Autodesk Inventor part; units mm, degrees
(part 2 of 2)
  line L281 (-95.3704, -44.7498) -> (-95.3704, -45.6606)
  spline S232 degree 2 poles (-95.3704, -45.6606) (-95.3704, -46.2246) (-95.539, -46.8665) (-95.6881, -47.0934) knots 0 0 0 1 2 2 2
  spline S233 degree 2 poles (-95.6881, -47.0934) (-95.9442, -47.4791) (-96.7902, -47.9037) (-97.3737, -47.9037) knots 0 0 0 1 2 2 2
  spline S234 degree 2 poles (-97.3672, -47.3494) (-96.9069, -47.3494) (-96.2553, -47.0447) (-96.0706, -46.7433) knots 0 0 0 1 2 2 2
  spline S235 degree 2 poles (-96.0706, -46.7433) (-95.9442, -46.5293) (-95.8307, -46.0464) (-95.8307, -45.6866) knots 0 0 0 1 2 2 2
  line L282 (-95.8307, -45.6866) -> (-95.8307, -45.2814)
  line L283 (-95.8307, -45.2814) -> (-98.9101, -45.2814)
  line L284 (-98.9101, -45.2814) -> (-98.9101, -45.6866)
  spline S236 degree 2 poles (-98.9101, -45.6866) (-98.9101, -46.0399) (-98.7967, -46.5747) (-98.6443, -46.7919) knots 0 0 0 1 2 2 2
  spline S237 degree 2 poles (-98.6443, -46.7919) (-98.4563, -47.0707) (-97.8339, -47.3494) (-97.3672, -47.3494) knots 0 0 0 1 2 2 2
  spline S238 degree 2 poles (-99.4385, -49.7449) (-99.4385, -49.0253) (-98.6314, -48.2344) (-97.8858, -48.2344) knots 0 0 0 1 2 2 2
  spline S239 degree 2 poles (-97.8858, -48.2344) (-97.1532, -48.2344) (-96.2845, -49.0026) (-96.2845, -49.6217) knots 0 0 0 1 2 2 2
  spline S240 degree 2 poles (-96.2845, -49.6217) (-96.2845, -49.9005) (-96.4466, -50.3316) (-96.6184, -50.4904) knots 0 0 0 1 2 2 2
  spline S241 degree 2 poles (-96.6184, -50.4904) (-96.7902, -50.6525) (-97.2861, -50.8243) (-97.6459, -50.8243) knots 0 0 0 1 2 2 2
  line L285 (-97.6459, -50.8243) -> (-97.9215, -50.8243)
  line L286 (-97.9215, -50.8243) -> (-97.9215, -48.7465)
  spline S242 degree 2 poles (-97.9215, -48.7465) (-98.4433, -48.7465) (-98.9976, -49.2716) (-98.9976, -49.7384) knots 0 0 0 1 2 2 2
  spline S243 degree 2 poles (-98.9976, -49.7384) (-98.9976, -49.9037) (-98.9231, -50.2246) (-98.8647, -50.3543) knots 0 0 0 1 2 2 2
  spline S244 degree 2 poles (-98.8647, -50.3543) (-98.7999, -50.4904) (-98.6865, -50.6784) (-98.6346, -50.74) knots 0 0 0 1 2 2 2
  line L287 (-98.6346, -50.74) -> (-98.6346, -50.7692)
  line L288 (-98.6346, -50.7692) -> (-99.1856, -50.7692)
  spline S245 degree 2 poles (-99.1856, -50.7692) (-99.2213, -50.6817) (-99.325, -50.4159) (-99.3542, -50.3122) knots 0 0 0 1 2 2 2
  spline S246 degree 2 poles (-99.3542, -50.3122) (-99.3963, -50.1663) (-99.4385, -49.9264) (-99.4385, -49.7449) knots 0 0 0 1 2 2 2
  spline S247 degree 2 poles (-97.5357, -50.3316) (-97.3315, -50.3251) (-97.0333, -50.2408) (-96.9328, -50.1598) knots 0 0 0 1 2 2 2
  spline S248 degree 2 poles (-96.9328, -50.1598) (-96.8194, -50.0723) (-96.6994, -49.7968) (-96.6994, -49.5926) knots 0 0 0 1 2 2 2
  spline S249 degree 2 poles (-96.6994, -49.5926) (-96.6994, -49.3916) (-96.8194, -49.1096) (-96.9361, -48.9929) knots 0 0 0 1 2 2 2
  spline S250 degree 2 poles (-96.9361, -48.9929) (-97.056, -48.8794) (-97.3445, -48.7627) (-97.5357, -48.7465) knots 0 0 0 1 2 2 2
  line L289 (-97.5357, -48.7465) -> (-97.5357, -50.3316)
  spline S251 degree 2 poles (-99.4417, -52.1468) (-99.4417, -51.8454) (-99.2797, -51.3235) (-99.1889, -51.1517) knots 0 0 0 1 2 2 2
  line L290 (-99.1889, -51.1517) -> (-98.6216, -51.1517)
  line L291 (-98.6216, -51.1517) -> (-98.6216, -51.1776)
  spline S252 degree 2 poles (-98.6216, -51.1776) (-98.6735, -51.2425) (-98.7967, -51.4175) (-98.8647, -51.5634) knots 0 0 0 1 2 2 2
  spline S253 degree 2 poles (-98.8647, -51.5634) (-98.9263, -51.6898) (-99.0171, -52.001) (-99.0171, -52.1663) knots 0 0 0 1 2 2 2
  spline S254 degree 2 poles (-99.0171, -52.1663) (-99.0171, -52.2862) (-98.962, -52.5618) (-98.9166, -52.6266) knots 0 0 0 1 2 2 2
  spline S255 degree 2 poles (-98.9166, -52.6266) (-98.855, -52.7206) (-98.7156, -52.8049) (-98.573, -52.8049) knots 0 0 0 1 2 2 2
  spline S256 degree 2 poles (-98.573, -52.8049) (-98.3947, -52.8049) (-98.21, -52.6104) (-98.1484, -52.3608) knots 0 0 0 1 2 2 2
  spline S257 degree 2 poles (-98.1484, -52.3608) (-98.1257, -52.2635) (-98.0609, -51.9524) (-98.0252, -51.8195) knots 0 0 0 1 2 2 2
  spline S258 degree 2 poles (-98.0252, -51.8195) (-97.9247, -51.4759) (-97.5098, -51.1647) (-97.2148, -51.1647) knots 0 0 0 1 2 2 2
  spline S259 degree 2 poles (-97.2148, -51.1647) (-96.8064, -51.1647) (-96.2975, -51.7773) (-96.2975, -52.283) knots 0 0 0 1 2 2 2
  spline S260 degree 2 poles (-96.2975, -52.283) (-96.2975, -52.5326) (-96.4207, -53.0383) (-96.5147, -53.2101) knots 0 0 0 1 2 2 2
  line L292 (-96.5147, -53.2101) -> (-97.056, -53.2101)
  line L293 (-97.056, -53.2101) -> (-97.056, -53.1841)
  spline S261 degree 2 poles (-97.056, -53.1841) (-96.9004, -52.9896) (-96.7221, -52.5164) (-96.7221, -52.2733) knots 0 0 0 1 2 2 2
  spline S262 degree 2 poles (-96.7221, -52.2733) (-96.7221, -52.0237) (-96.9328, -51.6801) (-97.1435, -51.6801) knots 0 0 0 1 2 2 2
  spline S263 degree 2 poles (-97.1435, -51.6801) (-97.3348, -51.6801) (-97.5195, -51.8843) (-97.5779, -52.1112) knots 0 0 0 1 2 2 2
  spline S264 degree 2 poles (-97.5779, -52.1112) (-97.607, -52.2214) (-97.6654, -52.5002) (-97.701, -52.6525) knots 0 0 0 1 2 2 2
  spline S265 degree 2 poles (-97.701, -52.6525) (-97.7853, -52.9831) (-98.1711, -53.3203) (-98.5049, -53.3203) knots 0 0 0 1 2 2 2
  spline S266 degree 2 poles (-98.5049, -53.3203) (-98.6994, -53.3203) (-99.043, -53.1679) (-99.1694, -53.0188) knots 0 0 0 1 2 2 2
  spline S267 degree 2 poles (-99.1694, -53.0188) (-99.3023, -52.86) (-99.4417, -52.4548) (-99.4417, -52.1468) knots 0 0 0 1 2 2 2
  line L294 (-99.3704, -54.3057) -> (-99.3704, -53.8)
  line L295 (-99.3704, -53.8) -> (-96.3688, -53.8)
  line L296 (-96.3688, -53.8) -> (-96.3688, -54.3057)
  line L297 (-96.3688, -54.3057) -> (-99.3704, -54.3057)
  line L298 (-95.8696, -54.3413) -> (-95.8696, -53.7676)
  line L299 (-95.8696, -53.7676) -> (-95.3445, -53.7676)
  line L300 (-95.3445, -53.7676) -> (-95.3445, -54.3413)
  line L301 (-95.3445, -54.3413) -> (-95.8696, -54.3413)
  spline S268 degree 2 poles (-99.8502, -55.1549) (-99.8728, -55.2068) (-99.9442, -55.4045) (-99.9733, -55.531) knots 0 0 0 1 2 2 2
  spline S269 degree 2 poles (-99.9733, -55.531) (-100.009, -55.6703) (-100.0511, -55.907) (-100.0511, -56.0464) knots 0 0 0 1 2 2 2
  spline S270 degree 2 poles (-100.0511, -56.0464) (-100.0511, -56.2797) (-99.9279, -56.6039) (-99.8177, -56.6947) knots 0 0 0 1 2 2 2
  spline S271 degree 2 poles (-99.8177, -56.6947) (-99.7075, -56.7822) (-99.419, -56.8502) (-99.2343, -56.8502) knots 0 0 0 1 2 2 2
  line L302 (-99.2343, -56.8502) -> (-98.9717, -56.8502)
  spline S272 degree 2 poles (-98.9717, -56.8502) (-99.15, -56.646) (-99.3185, -56.2538) (-99.3185, -55.9588) knots 0 0 0 1 2 2 2
  spline S273 degree 2 poles (-99.3185, -55.9588) (-99.3185, -55.4467) (-98.5568, -54.8405) (-97.8404, -54.8405) knots 0 0 0 1 2 2 2
  spline S274 degree 2 poles (-97.8404, -54.8405) (-97.4677, -54.8405) (-96.8907, -55.0512) (-96.6865, -55.2263) knots 0 0 0 1 2 2 2
  spline S275 degree 2 poles (-96.6865, -55.2263) (-96.4952, -55.3948) (-96.2845, -55.8584) (-96.2845, -56.1047) knots 0 0 0 1 2 2 2
  spline S276 degree 2 poles (-96.2845, -56.1047) (-96.2845, -56.3381) (-96.3947, -56.6784) (-96.4952, -56.8502) knots 0 0 0 1 2 2 2
  line L303 (-96.4952, -56.8502) -> (-96.3688, -56.8794)
  line L304 (-96.3688, -56.8794) -> (-96.3688, -57.3559)
  line L305 (-96.3688, -57.3559) -> (-99.0268, -57.3559)
  spline S277 degree 2 poles (-99.0268, -57.3559) (-99.7918, -57.3559) (-100.5049, -56.6914) (-100.5049, -56.0075) knots 0 0 0 1 2 2 2
  spline S278 degree 2 poles (-100.5049, -56.0075) (-100.5049, -55.787) (-100.4336, -55.3267) (-100.3753, -55.129) knots 0 0 0 1 2 2 2
  line L306 (-100.3753, -55.129) -> (-99.8502, -55.129)
  line L307 (-99.8502, -55.129) -> (-99.8502, -55.1549)
  line L308 (-98.5568, -56.8502) -> (-96.9069, -56.8502)
  spline S279 degree 2 poles (-96.9069, -56.8502) (-96.8161, -56.6622) (-96.7383, -56.3446) (-96.7383, -56.1857) knots 0 0 0 1 2 2 2
  spline S280 degree 2 poles (-96.7383, -56.1857) (-96.7383, -55.8032) (-97.3023, -55.3624) (-97.8307, -55.3624) knots 0 0 0 1 2 2 2
  spline S281 degree 2 poles (-97.8307, -55.3624) (-98.3299, -55.3624) (-98.8518, -55.6963) (-98.8518, -56.0723) knots 0 0 0 1 2 2 2
  spline S282 degree 2 poles (-98.8518, -56.0723) (-98.8518, -56.27) (-98.6962, -56.6849) (-98.5568, -56.8502) knots 0 0 0 1 2 2 2
  line L309 (-99.3704, -60.4451) -> (-99.3704, -59.9394)
  line L310 (-99.3704, -59.9394) -> (-97.6589, -59.9394)
  spline S283 degree 2 poles (-97.6589, -59.9394) (-97.4514, -59.9394) (-97.0949, -59.9005) (-96.9879, -59.8421) knots 0 0 0 1 2 2 2
  spline S284 degree 2 poles (-96.9879, -59.8421) (-96.8745, -59.7806) (-96.7643, -59.5601) (-96.7643, -59.3721) knots 0 0 0 1 2 2 2
  spline S285 degree 2 poles (-96.7643, -59.3721) (-96.7643, -59.1841) (-96.9652, -58.7854) (-97.1273, -58.5942) knots 0 0 0 1 2 2 2
  line L311 (-97.1273, -58.5942) -> (-99.3704, -58.5942)
  line L312 (-99.3704, -58.5942) -> (-99.3704, -58.0885)
  line L313 (-99.3704, -58.0885) -> (-96.3688, -58.0885)
  line L314 (-96.3688, -58.0885) -> (-96.3688, -58.5942)
  line L315 (-96.3688, -58.5942) -> (-96.7027, -58.5942)
  spline S286 degree 2 poles (-96.7027, -58.5942) (-96.4985, -58.8211) (-96.2845, -59.2587) (-96.2845, -59.505) knots 0 0 0 1 2 2 2
  spline S287 degree 2 poles (-96.2845, -59.505) (-96.2845, -59.9459) (-96.868, -60.4451) (-97.4223, -60.4451) knots 0 0 0 1 2 2 2
  line L316 (-97.4223, -60.4451) -> (-99.3704, -60.4451)
  spline S288 degree 2 poles (-98.1419, -65.625) (-98.4401, -65.625) (-98.8972, -65.3981) (-99.0463, -65.2101) knots 0 0 0 1 2 2 2
  spline S289 degree 2 poles (-99.0463, -65.2101) (-99.2213, -64.9831) (-99.3704, -64.4678) (-99.3704, -64.0593) knots 0 0 0 1 2 2 2
  line L317 (-99.3704, -64.0593) -> (-99.3704, -62.9118)
  line L318 (-99.3704, -62.9118) -> (-95.3704, -62.9118)
  line L319 (-95.3704, -62.9118) -> (-95.3704, -63.9718)
  spline S290 degree 2 poles (-95.3704, -63.9718) (-95.3704, -64.3997) (-95.4255, -64.8276) (-95.5325, -65.022) knots 0 0 0 1 2 2 2
  spline S291 degree 2 poles (-95.5325, -65.022) (-95.6459, -65.2392) (-96.0187, -65.437) (-96.2715, -65.437) knots 0 0 0 1 2 2 2
  spline S292 degree 2 poles (-96.2715, -65.437) (-96.5536, -65.437) (-97.0009, -65.1387) (-97.1273, -64.8762) knots 0 0 0 1 2 2 2
  line L320 (-97.1273, -64.8762) -> (-97.1467, -64.8762)
  spline S293 degree 2 poles (-97.1467, -64.8762) (-97.244, -65.2327) (-97.7594, -65.625) (-98.1419, -65.625) knots 0 0 0 1 2 2 2
  spline S294 degree 2 poles (-98.1646, -65.0707) (-97.9377, -65.0707) (-97.6459, -64.941) (-97.5422, -64.7465) knots 0 0 0 1 2 2 2
  spline S295 degree 2 poles (-97.5422, -64.7465) (-97.4774, -64.6201) (-97.4385, -64.3219) (-97.4385, -64.0464) knots 0 0 0 1 2 2 2
  line L321 (-97.4385, -64.0464) -> (-97.4385, -63.4434)
  line L322 (-97.4385, -63.4434) -> (-98.9166, -63.4434)
  line L323 (-98.9166, -63.4434) -> (-98.9166, -63.8746)
  spline S296 degree 2 poles (-98.9166, -63.8746) (-98.9166, -64.2246) (-98.8518, -64.6266) (-98.748, -64.7822) knots 0 0 0 1 2 2 2
  spline S297 degree 2 poles (-98.748, -64.7822) (-98.6411, -64.9313) (-98.3753, -65.0707) (-98.1646, -65.0707) knots 0 0 0 1 2 2 2
  spline S298 degree 2 poles (-96.3461, -64.8827) (-96.2035, -64.8827) (-95.9895, -64.7854) (-95.9279, -64.6784) knots 0 0 0 1 2 2 2
  spline S299 degree 2 poles (-95.9279, -64.6784) (-95.8566, -64.5488) (-95.8242, -64.2344) (-95.8242, -63.9524) knots 0 0 0 1 2 2 2
  line L324 (-95.8242, -63.9524) -> (-95.8242, -63.4434)
  line L325 (-95.8242, -63.4434) -> (-96.9944, -63.4434)
  line L326 (-96.9944, -63.4434) -> (-96.9944, -64.0464)
  spline S300 degree 2 poles (-96.9944, -64.0464) (-96.9944, -64.296) (-96.9425, -64.5326) (-96.8615, -64.659) knots 0 0 0 1 2 2 2
  spline S301 degree 2 poles (-96.8615, -64.659) (-96.7837, -64.7822) (-96.5341, -64.8827) (-96.3461, -64.8827) knots 0 0 0 1 2 2 2
  line L327 (-96.3688, -68.471) -> (-100.4758, -66.8567)
  line L328 (-100.4758, -66.8567) -> (-100.4758, -66.3154)
  line L329 (-100.4758, -66.3154) -> (-99.2245, -66.8535)
  line L330 (-99.2245, -66.8535) -> (-96.3688, -65.7643)
  line L331 (-96.3688, -65.7643) -> (-96.3688, -66.3089)
  line L332 (-96.3688, -66.3089) -> (-98.5925, -67.129)
  line L333 (-98.5925, -67.129) -> (-96.3688, -67.9459)
  line L334 (-96.3688, -67.9459) -> (-96.3688, -68.471)
  line L335 (-99.3704, -69.7806) -> (-99.3704, -69.1387)
  line L336 (-99.3704, -69.1387) -> (-98.6054, -69.1387)
  line L337 (-98.6054, -69.1387) -> (-98.6054, -69.7806)
  line L338 (-98.6054, -69.7806) -> (-99.3704, -69.7806)
  line L339 (-97.1338, -69.7806) -> (-97.1338, -69.1387)
  line L340 (-97.1338, -69.1387) -> (-96.3688, -69.1387)
  line L341 (-96.3688, -69.1387) -> (-96.3688, -69.7806)
  line L342 (-96.3688, -69.7806) -> (-97.1338, -69.7806)
  line L343 (-109.2392, -46.2221) -> (-109.2392, -44.2853)
  line L344 (-109.2392, -44.2853) -> (-108.7287, -44.2853)
  line L345 (-108.7287, -44.2853) -> (-108.7287, -44.9215)
  line L346 (-108.7287, -44.9215) -> (-104.7498, -44.9215)
  line L347 (-104.7498, -44.9215) -> (-104.7498, -44.2853)
  line L348 (-104.7498, -44.2853) -> (-104.2392, -44.2853)
  line L349 (-104.2392, -44.2853) -> (-104.2392, -46.2221)
  line L350 (-104.2392, -46.2221) -> (-104.7498, -46.2221)
  line L351 (-104.7498, -46.2221) -> (-104.7498, -45.586)
  line L352 (-104.7498, -45.586) -> (-108.7287, -45.586)
  line L353 (-108.7287, -45.586) -> (-108.7287, -46.2221)
  line L354 (-108.7287, -46.2221) -> (-109.2392, -46.2221)
  line L355 (-109.2392, -51.2505) -> (-107.0674, -51.2505)
  spline S302 degree 2 poles (-107.0674, -51.2505) (-106.8081, -51.2505) (-106.3665, -51.21) (-106.2449, -51.1451) knots 0 0 0 1 2 2 2
  spline S303 degree 2 poles (-106.2449, -51.1451) (-106.1112, -51.0803) (-105.9815, -50.8331) (-105.9815, -50.6184) knots 0 0 0 1 2 2 2
  spline S304 degree 2 poles (-105.9815, -50.6184) (-105.9815, -50.4239) (-106.2206, -49.9782) (-106.4475, -49.7432) knots 0 0 0 1 2 2 2
  spline S305 degree 2 poles (-106.4475, -49.7432) (-106.5042, -49.7472) (-106.6622, -49.7553) (-106.7676, -49.7553) knots 0 0 0 1 2 2 2
  line L356 (-106.7676, -49.7553) -> (-109.2392, -49.7553)
  line L357 (-109.2392, -49.7553) -> (-109.2392, -49.1232)
  line L358 (-109.2392, -49.1232) -> (-107.0674, -49.1232)
  spline S306 degree 2 poles (-107.0674, -49.1232) (-106.8081, -49.1232) (-106.3665, -49.0827) (-106.2449, -49.0179) knots 0 0 0 1 2 2 2
  spline S307 degree 2 poles (-106.2449, -49.0179) (-106.1112, -48.9531) (-105.9815, -48.7059) (-105.9815, -48.4912) knots 0 0 0 1 2 2 2
  spline S308 degree 2 poles (-105.9815, -48.4912) (-105.9815, -48.2886) (-106.2368, -47.8388) (-106.4353, -47.6281) knots 0 0 0 1 2 2 2
  line L359 (-106.4353, -47.6281) -> (-109.2392, -47.6281)
  line L360 (-109.2392, -47.6281) -> (-109.2392, -46.996)
  line L361 (-109.2392, -46.996) -> (-105.4872, -46.996)
  line L362 (-105.4872, -46.996) -> (-105.4872, -47.6281)
  line L363 (-105.4872, -47.6281) -> (-105.9005, -47.6281)
  spline S309 degree 2 poles (-105.9005, -47.6281) (-105.6533, -47.8753) (-105.3819, -48.3615) (-105.3819, -48.6532) knots 0 0 0 1 2 2 2
  spline S310 degree 2 poles (-105.3819, -48.6532) (-105.3819, -48.9855) (-105.6857, -49.5001) (-106.0302, -49.6338) knots 0 0 0 1 2 2 2
  spline S311 degree 2 poles (-106.0302, -49.6338) (-105.7101, -49.9215) (-105.3819, -50.4644) (-105.3819, -50.7805) knots 0 0 0 1 2 2 2
  spline S312 degree 2 poles (-105.3819, -50.7805) (-105.3819, -51.0236) (-105.5318, -51.4207) (-105.702, -51.5665) knots 0 0 0 1 2 2 2
  spline S313 degree 2 poles (-105.702, -51.5665) (-105.8721, -51.7164) (-106.3827, -51.8826) (-106.7676, -51.8826) knots 0 0 0 1 2 2 2
  line L364 (-106.7676, -51.8826) -> (-109.2392, -51.8826)
  line L365 (-109.2392, -51.8826) -> (-109.2392, -51.2505)
  spline S314 degree 2 poles (-107.3632, -55.8534) (-108.3114, -55.8534) (-109.3446, -54.9417) (-109.3446, -54.18) knots 0 0 0 1 2 2 2
  spline S315 degree 2 poles (-109.3446, -54.18) (-109.3446, -53.398) (-108.2789, -52.5025) (-107.3632, -52.5025) knots 0 0 0 1 2 2 2
  spline S316 degree 2 poles (-107.3632, -52.5025) (-106.4232, -52.5025) (-105.3819, -53.4263) (-105.3819, -54.18) knots 0 0 0 1 2 2 2
  spline S317 degree 2 poles (-105.3819, -54.18) (-105.3819, -54.9417) (-106.4191, -55.8534) (-107.3632, -55.8534) knots 0 0 0 1 2 2 2
  spline S318 degree 2 poles (-107.3632, -55.201) (-106.6339, -55.201) (-105.9248, -54.6703) (-105.9248, -54.18) knots 0 0 0 1 2 2 2
  spline S319 degree 2 poles (-105.9248, -54.18) (-105.9248, -53.6897) (-106.6339, -53.1549) (-107.3632, -53.1549) knots 0 0 0 1 2 2 2
  spline S320 degree 2 poles (-107.3632, -53.1549) (-108.0723, -53.1549) (-108.8016, -53.6897) (-108.8016, -54.18) knots 0 0 0 1 2 2 2
  spline S321 degree 2 poles (-108.8016, -54.18) (-108.8016, -54.6662) (-108.0845, -55.201) (-107.3632, -55.201) knots 0 0 0 1 2 2 2
  spline S322 degree 2 poles (-109.8389, -56.6354) (-109.8673, -56.7002) (-109.9564, -56.9474) (-109.9929, -57.1054) knots 0 0 0 1 2 2 2
  spline S323 degree 2 poles (-109.9929, -57.1054) (-110.0375, -57.2797) (-110.0901, -57.5754) (-110.0901, -57.7497) knots 0 0 0 1 2 2 2
  spline S324 degree 2 poles (-110.0901, -57.7497) (-110.0901, -58.0414) (-109.9362, -58.4466) (-109.7984, -58.56) knots 0 0 0 1 2 2 2
  spline S325 degree 2 poles (-109.7984, -58.56) (-109.6606, -58.6694) (-109.3, -58.7545) (-109.0691, -58.7545) knots 0 0 0 1 2 2 2
  line L366 (-109.0691, -58.7545) -> (-108.7409, -58.7545)
  spline S326 degree 2 poles (-108.7409, -58.7545) (-108.9637, -58.4993) (-109.1744, -58.009) (-109.1744, -57.6403) knots 0 0 0 1 2 2 2
  spline S327 degree 2 poles (-109.1744, -57.6403) (-109.1744, -57.0001) (-108.2222, -56.2424) (-107.3268, -56.2424) knots 0 0 0 1 2 2 2
  spline S328 degree 2 poles (-107.3268, -56.2424) (-106.8608, -56.2424) (-106.1396, -56.5057) (-105.8843, -56.7245) knots 0 0 0 1 2 2 2
  spline S329 degree 2 poles (-105.8843, -56.7245) (-105.6452, -56.9352) (-105.3819, -57.5147) (-105.3819, -57.8226) knots 0 0 0 1 2 2 2
  spline S330 degree 2 poles (-105.3819, -57.8226) (-105.3819, -58.1143) (-105.5196, -58.5398) (-105.6452, -58.7545) knots 0 0 0 1 2 2 2
  line L367 (-105.6452, -58.7545) -> (-105.4872, -58.791)
  line L368 (-105.4872, -58.791) -> (-105.4872, -59.3866)
  line L369 (-105.4872, -59.3866) -> (-108.8097, -59.3866)
  spline S331 degree 2 poles (-108.8097, -59.3866) (-109.766, -59.3866) (-110.6574, -58.556) (-110.6574, -57.701) knots 0 0 0 1 2 2 2
  spline S332 degree 2 poles (-110.6574, -57.701) (-110.6574, -57.4255) (-110.5682, -56.8502) (-110.4953, -56.603) knots 0 0 0 1 2 2 2
  line L370 (-110.4953, -56.603) -> (-109.8389, -56.603)
  line L371 (-109.8389, -56.603) -> (-109.8389, -56.6354)
  line L372 (-108.2222, -58.7545) -> (-106.1598, -58.7545)
  spline S333 degree 2 poles (-106.1598, -58.7545) (-106.0464, -58.5195) (-105.9491, -58.1224) (-105.9491, -57.9239) knots 0 0 0 1 2 2 2
  spline S334 degree 2 poles (-105.9491, -57.9239) (-105.9491, -57.4458) (-106.6541, -56.8947) (-107.3146, -56.8947) knots 0 0 0 1 2 2 2
  spline S335 degree 2 poles (-107.3146, -56.8947) (-107.9386, -56.8947) (-108.5909, -57.3121) (-108.5909, -57.7821) knots 0 0 0 1 2 2 2
  spline S336 degree 2 poles (-108.5909, -57.7821) (-108.5909, -58.0292) (-108.3964, -58.5479) (-108.2222, -58.7545) knots 0 0 0 1 2 2 2
  spline S337 degree 2 poles (-109.3243, -61.9312) (-109.3243, -61.0317) (-108.3154, -60.043) (-107.3835, -60.043) knots 0 0 0 1 2 2 2
  spline S338 degree 2 poles (-107.3835, -60.043) (-106.4678, -60.043) (-105.3819, -61.0033) (-105.3819, -61.7772) knots 0 0 0 1 2 2 2
  spline S339 degree 2 poles (-105.3819, -61.7772) (-105.3819, -62.1257) (-105.5845, -62.6646) (-105.7992, -62.8631) knots 0 0 0 1 2 2 2
  spline S340 degree 2 poles (-105.7992, -62.8631) (-106.014, -63.0657) (-106.6339, -63.2805) (-107.0836, -63.2805) knots 0 0 0 1 2 2 2
  line L373 (-107.0836, -63.2805) -> (-107.4281, -63.2805)
  line L374 (-107.4281, -63.2805) -> (-107.4281, -60.6832)
  spline S341 degree 2 poles (-107.4281, -60.6832) (-108.0804, -60.6832) (-108.7733, -61.3396) (-108.7733, -61.9231) knots 0 0 0 1 2 2 2
  spline S342 degree 2 poles (-108.7733, -61.9231) (-108.7733, -62.1297) (-108.6801, -62.5309) (-108.6071, -62.6929) knots 0 0 0 1 2 2 2
  spline S343 degree 2 poles (-108.6071, -62.6929) (-108.5261, -62.8631) (-108.3843, -63.0981) (-108.3195, -63.1751) knots 0 0 0 1 2 2 2
  line L375 (-108.3195, -63.1751) -> (-108.3195, -63.2116)
  line L376 (-108.3195, -63.2116) -> (-109.0083, -63.2116)
  spline S344 degree 2 poles (-109.0083, -63.2116) (-109.0528, -63.1022) (-109.1825, -62.7699) (-109.219, -62.6403) knots 0 0 0 1 2 2 2
  spline S345 degree 2 poles (-109.219, -62.6403) (-109.2716, -62.4579) (-109.3243, -62.1581) (-109.3243, -61.9312) knots 0 0 0 1 2 2 2
  spline S346 degree 2 poles (-106.9459, -62.6646) (-106.6906, -62.6565) (-106.3178, -62.5511) (-106.1922, -62.4498) knots 0 0 0 1 2 2 2
  spline S347 degree 2 poles (-106.1922, -62.4498) (-106.0504, -62.3404) (-105.9005, -61.996) (-105.9005, -61.7408) knots 0 0 0 1 2 2 2
  spline S348 degree 2 poles (-105.9005, -61.7408) (-105.9005, -61.4895) (-106.0504, -61.137) (-106.1963, -60.9912) knots 0 0 0 1 2 2 2
  spline S349 degree 2 poles (-106.1963, -60.9912) (-106.3462, -60.8493) (-106.7068, -60.7035) (-106.9459, -60.6832) knots 0 0 0 1 2 2 2
  line L377 (-106.9459, -60.6832) -> (-106.9459, -62.6646)
  line L378 (-109.2392, -66.8664) -> (-109.2392, -66.2343)
  line L379 (-109.2392, -66.2343) -> (-107.0999, -66.2343)
  spline S350 degree 2 poles (-107.0999, -66.2343) (-106.8405, -66.2343) (-106.3948, -66.1856) (-106.2611, -66.1127) knots 0 0 0 1 2 2 2
  spline S351 degree 2 poles (-106.2611, -66.1127) (-106.1193, -66.0357) (-105.9815, -65.7602) (-105.9815, -65.5252) knots 0 0 0 1 2 2 2
  spline S352 degree 2 poles (-105.9815, -65.5252) (-105.9815, -65.2902) (-106.2328, -64.7918) (-106.4353, -64.5527) knots 0 0 0 1 2 2 2
  line L380 (-106.4353, -64.5527) -> (-109.2392, -64.5527)
  line L381 (-109.2392, -64.5527) -> (-109.2392, -63.9207)
  line L382 (-109.2392, -63.9207) -> (-105.4872, -63.9207)
  line L383 (-105.4872, -63.9207) -> (-105.4872, -64.5527)
  line L384 (-105.4872, -64.5527) -> (-105.9046, -64.5527)
  spline S353 degree 2 poles (-105.9046, -64.5527) (-105.6493, -64.8364) (-105.3819, -65.3834) (-105.3819, -65.6913) knots 0 0 0 1 2 2 2
  spline S354 degree 2 poles (-105.3819, -65.6913) (-105.3819, -66.2424) (-106.1112, -66.8664) (-106.8041, -66.8664) knots 0 0 0 1 2 2 2
  line L385 (-106.8041, -66.8664) -> (-109.2392, -66.8664)
  line L386 (-104.2392, -75.5536) -> (-109.2392, -74.2975)
  line L387 (-109.2392, -74.2975) -> (-109.2392, -73.5519)
  line L388 (-109.2392, -73.5519) -> (-105.0901, -72.5349)
  line L389 (-105.0901, -72.5349) -> (-109.2392, -71.5463)
  line L390 (-109.2392, -71.5463) -> (-109.2392, -70.8088)
  line L391 (-109.2392, -70.8088) -> (-104.2392, -69.5325)
  line L392 (-104.2392, -69.5325) -> (-104.2392, -70.2173)
  line L393 (-104.2392, -70.2173) -> (-108.3843, -71.2221)
  line L394 (-108.3843, -71.2221) -> (-104.2392, -72.2189)
  line L395 (-104.2392, -72.2189) -> (-104.2392, -72.8955)
  line L396 (-104.2392, -72.8955) -> (-108.4329, -73.9004)
  line L397 (-108.4329, -73.9004) -> (-104.2392, -74.9012)
  line L398 (-104.2392, -74.9012) -> (-104.2392, -75.5536)
  line L399 (-106.1639, -78.09) -> (-106.1639, -78.0576)
  spline S355 degree 2 poles (-106.1639, -78.0576) (-106.1436, -77.9847) (-106.1355, -77.8267) (-106.1355, -77.7173) knots 0 0 0 1 2 2 2
  spline S356 degree 2 poles (-106.1355, -77.7173) (-106.1355, -77.462) (-106.3584, -76.9596) (-106.5772, -76.7326) knots 0 0 0 1 2 2 2
  line L400 (-106.5772, -76.7326) -> (-109.2392, -76.7326)
  line L401 (-109.2392, -76.7326) -> (-109.2392, -76.1006)
  line L402 (-109.2392, -76.1006) -> (-105.4872, -76.1006)
  line L403 (-105.4872, -76.1006) -> (-105.4872, -76.7326)
  line L404 (-105.4872, -76.7326) -> (-106.0464, -76.7326)
  spline S357 degree 2 poles (-106.0464, -76.7326) (-105.7384, -77.0771) (-105.4872, -77.5916) (-105.4872, -77.8348) knots 0 0 0 1 2 2 2
  spline S358 degree 2 poles (-105.4872, -77.8348) (-105.4872, -77.932) (-105.4953, -78.0292) (-105.5075, -78.09) knots 0 0 0 1 2 2 2
  line L405 (-105.5075, -78.09) -> (-106.1639, -78.09)
  spline S359 degree 2 poles (-109.3243, -80.2091) (-109.3243, -79.3096) (-108.3154, -78.321) (-107.3835, -78.321) knots 0 0 0 1 2 2 2
  spline S360 degree 2 poles (-107.3835, -78.321) (-106.4678, -78.321) (-105.3819, -79.2813) (-105.3819, -80.0552) knots 0 0 0 1 2 2 2
  spline S361 degree 2 poles (-105.3819, -80.0552) (-105.3819, -80.4036) (-105.5845, -80.9425) (-105.7992, -81.1411) knots 0 0 0 1 2 2 2
  spline S362 degree 2 poles (-105.7992, -81.1411) (-106.014, -81.3437) (-106.6339, -81.5584) (-107.0836, -81.5584) knots 0 0 0 1 2 2 2
  line L406 (-107.0836, -81.5584) -> (-107.4281, -81.5584)
  line L407 (-107.4281, -81.5584) -> (-107.4281, -78.9612)
  spline S363 degree 2 poles (-107.4281, -78.9612) (-108.0804, -78.9612) (-108.7733, -79.6176) (-108.7733, -80.201) knots 0 0 0 1 2 2 2
  spline S364 degree 2 poles (-108.7733, -80.201) (-108.7733, -80.4077) (-108.6801, -80.8088) (-108.6071, -80.9709) knots 0 0 0 1 2 2 2
  spline S365 degree 2 poles (-108.6071, -80.9709) (-108.5261, -81.1411) (-108.3843, -81.3761) (-108.3195, -81.4531) knots 0 0 0 1 2 2 2
  line L408 (-108.3195, -81.4531) -> (-108.3195, -81.4895)
  line L409 (-108.3195, -81.4895) -> (-109.0083, -81.4895)
  spline S366 degree 2 poles (-109.0083, -81.4895) (-109.0528, -81.3801) (-109.1825, -81.0479) (-109.219, -80.9182) knots 0 0 0 1 2 2 2
  spline S367 degree 2 poles (-109.219, -80.9182) (-109.2716, -80.7359) (-109.3243, -80.4361) (-109.3243, -80.2091) knots 0 0 0 1 2 2 2
  spline S368 degree 2 poles (-106.9459, -80.9425) (-106.6906, -80.9344) (-106.3178, -80.8291) (-106.1922, -80.7278) knots 0 0 0 1 2 2 2
  spline S369 degree 2 poles (-106.1922, -80.7278) (-106.0504, -80.6184) (-105.9005, -80.274) (-105.9005, -80.0187) knots 0 0 0 1 2 2 2
  spline S370 degree 2 poles (-105.9005, -80.0187) (-105.9005, -79.7675) (-106.0504, -79.415) (-106.1963, -79.2691) knots 0 0 0 1 2 2 2
  spline S371 degree 2 poles (-106.1963, -79.2691) (-106.3462, -79.1273) (-106.7068, -78.9814) (-106.9459, -78.9612) knots 0 0 0 1 2 2 2
  line L410 (-106.9459, -78.9612) -> (-106.9459, -80.9425)
  line L411 (-109.2392, -85.1443) -> (-109.2392, -84.5122)
  line L412 (-109.2392, -84.5122) -> (-107.0999, -84.5122)
  spline S372 degree 2 poles (-107.0999, -84.5122) (-106.8405, -84.5122) (-106.3948, -84.4636) (-106.2611, -84.3907) knots 0 0 0 1 2 2 2
  spline S373 degree 2 poles (-106.2611, -84.3907) (-106.1193, -84.3137) (-105.9815, -84.0382) (-105.9815, -83.8032) knots 0 0 0 1 2 2 2
  spline S374 degree 2 poles (-105.9815, -83.8032) (-105.9815, -83.5681) (-106.2328, -83.0698) (-106.4353, -82.8307) knots 0 0 0 1 2 2 2
  line L413 (-106.4353, -82.8307) -> (-109.2392, -82.8307)
  line L414 (-109.2392, -82.8307) -> (-109.2392, -82.1986)
  line L415 (-109.2392, -82.1986) -> (-105.4872, -82.1986)
  line L416 (-105.4872, -82.1986) -> (-105.4872, -82.8307)
  line L417 (-105.4872, -82.8307) -> (-105.9046, -82.8307)
  spline S375 degree 2 poles (-105.9046, -82.8307) (-105.6493, -83.1143) (-105.3819, -83.6613) (-105.3819, -83.9693) knots 0 0 0 1 2 2 2
  spline S376 degree 2 poles (-105.3819, -83.9693) (-105.3819, -84.5203) (-106.1112, -85.1443) (-106.8041, -85.1443) knots 0 0 0 1 2 2 2
  line L418 (-106.8041, -85.1443) -> (-109.2392, -85.1443)
  point P0 (0, 0)
  constraints: 12 other
chamfer "Chamfer1" distance 10 angle 45 2 edges at (-87.4562, 74.4586, -1.5) (-92.5687, -88.3406, -1.5)
extrude "Extrusion2" cut sketch "Sketch2" against normal blind 2
body "Solid1"
